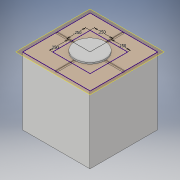
# Autodesk Inventor part: companion_cube
Saved by Autodesk Inventor 2017 (Build 210142000, 142)
## iProperties
Created: 2018-10-23
Part Number: companion_cube
Material: Generic
Document SubType Name: Modeling
Designer: jacob
Density: 1 g/cm^3
Appearance: Default
Author: jacob
Autodesk Inventor part; units mm, degrees
ref_plane "YZ Plane" through (0, 0, 0) normal (1, 0, 0) x (0, 1, 0)
ref_plane "XY Plane" through (0, 0, 0) normal (0, 0, 1) x (1, 0, 0)
sketch "Sketch1" plane through (0, 0, 0) normal (0, 1, 0) x (-1, 0, 0)
  line L0 (11.43, 11.43) -> (-11.43, 11.43)
  line L1 (-11.43, 11.43) -> (-11.43, -11.43)
  line L2 (-11.43, -11.43) -> (11.43, -11.43)
  line L3 (11.43, -11.43) -> (11.43, 11.43)
  line L4 (0.381, -11.43) -> (0.381, 11.43)
  line L5 (-0.381, -11.43) -> (-0.381, 11.43)
  line L6 (11.43, -0.381) -> (-11.43, -0.381)
  line L7 (11.43, 0.381) -> (-11.43, 0.381)
  circle A0 centre (0, 0) radius 5.08
  dimension "d0" = 22.86
  dimension "d1" = 22.86
  dimension "d2" = 11.43
  dimension "d3" = 11.43
  dimension "d7" = 0.381
  dimension "d8" = 0.762
  dimension "d12" = 0.381
  dimension "d13" = 0.381
  dimension "d14" = 0.762
  dimension "d21" = 10.16
  constraints: 16 end point, 8 point on line, 5 perpendicular, 2 parallel, 1 centre point, 1 coincident, 1 horizontal
  measures "d0" distance of L2.end L0.start
  measures "d1" distance of L1.end L2.end
  measures "d2" distance from line of point (0, 0) L0
  measures "d3" distance from line of point (0, 0) L3
  measures "d7" distance from line of point (0, 0) L4
  measures "d8" distance between parallel lines of L4 L5
  measures "d12" distance from line of point (0, 0) L6
  measures "d13" distance from line of point (0, 0) L7
  measures "d14" distance between parallel lines of L7 L6
  measures "d21" diameter of A0
extrude "Extrusion2" add sketch "Sketch1" against normal blind 22.86
extrude "Extrusion3" cut sketch "Sketch1" against normal blind 0.254 contours L4 A0 L5 L0 | L3 L6 A0 L7 | L4 L7 L5 A0 | A0 L6 L4 L7 | L4 L6 L5 L7 | L7 A0 L6 L1 | L5 L6 A0 L7 | L4 A0 L5 L6 | L2 L5 A0 L4
extrude "Extrusion4" add sketch "Sketch1" along normal blind 0.508 contours A0 L7 L4 | L4 L7 L5 A0 | A0 L6 L4 L7 | L5 L7 A0 | L4 L6 L5 L7 | A0 L4 L6 | L5 L6 A0 L7 | L4 A0 L5 L6 | L5 A0 L6
sketch "Sketch2" plane through (0, 0, 0) normal (0, 1, 0) x (-1, 0, 0)
  line L0 (0.381, -11.43) -> (11.43, -11.43) projected
  line L1 (-0.381, 11.43) -> (-11.43, 11.43) projected
  line L2 (11.43, -11.43) -> (-11.43, -11.43)
  line L3 (-11.43, -11.43) -> (-11.43, 11.43)
  line L4 (-11.43, 11.43) -> (11.43, 11.43)
  line L5 (11.43, 11.43) -> (11.43, -11.43)
  line L6 (6.35, -6.35) -> (-6.35, -6.35)
  line L7 (-6.35, -6.35) -> (-6.35, 6.35)
  line L8 (-6.35, 6.35) -> (6.35, 6.35)
  line L9 (6.35, 6.35) -> (6.35, -6.35)
  point P0 (0, 0)
  dimension "d24" = 6.35
  dimension "d25" = 6.35
  dimension "d26" = 6.35
  dimension "d27" = 6.35
  constraints: 16 end point, 4 parallel, 2 horizontal, 2 perpendicular
  measures "d24" distance from line of point (0, 0) L9
  measures "d25" distance from line of point (0, 0) L7
  measures "d26" distance from line of point (0, 0) L6
  measures "d27" distance from line of point (0, 0) L8
body "Solid2"
